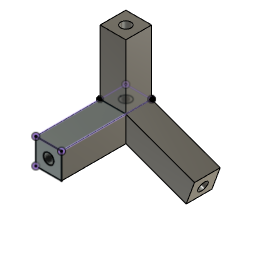
Collin_Corner Connector 2 v1 v1 (Autodesk Fusion 360 design; units mm, degrees)
Autodesk Fusion 360 part; units mm, degrees
sketch "Sketch1" plane through (0, 0, 0) normal (0, 1, 0) x (1, 0, 0)
  line L0 (0, 0) -> (4, 0)
  line L1 (4, 0) -> (4, -4)
  line L2 (4, -4) -> (0, -4)
  line L3 (0, -4) -> (0, 0)
  circle A0 centre (2, -2) radius 0.8
  dimension "d1" = 4
  dimension "d2" = 4
  dimension "d3" = 1.6
  dimension "d4" = 2
  dimension "d5" = 2
  constraint horizontal L0
  constraint vertical L1
  constraint horizontal L2
  constraint vertical L3
  constraint coincident L0.start L3.end
  measures "d1" distance of L1.end L2.end
  measures "d2" distance of L0.end L1.end
  measures "d3" diameter of A0
  measures "d4" distance of L2 A0.centre
  measures "d5" distance of L1 A0.centre
extrude "Extrude1" add sketch "Sketch1" along normal blind 14 makes body 1
sketch "Sketch2" plane through (0, 0, 4) normal (0, 0, 1) x (-1, 0, 0)
  line L0 (0, 0) -> (-4, 0)
  line L1 (-4, 0) -> (-4, -14)
  line L2 (-4, -14) -> (0, -14)
  line L3 (0, -14) -> (0, 0)
  line L4 (-4, -14) -> (0, -14)
  line L5 (0, -14) -> (0, -10)
  line L6 (0, -10) -> (-4, -10)
  line L7 (-4, -10) -> (-4, -14)
  circle A0 centre (-2, -12) radius 0.8
  dimension "d8" = 4
  dimension "d9" = 1.6
  dimension "d10" = 2
  dimension "d11" = 2
  constraint horizontal L4
  constraint vertical L5
  constraint horizontal L6
  constraint vertical L7
  constraint coincident L3 L5.end
  constraint coincident L1.end L2.start
  measures "d8" distance of L4 L6
  measures "d9" diameter of A0
  measures "d10" distance of L5 A0.centre
  measures "d11" distance of L4 A0.centre
extrude "Extrude2" add sketch "Sketch2" along normal blind 10 contours L1 L2 L3 L4 L5 L6 L7 bodies 1
ref_plane "WorkPlane1" through (4, 7, 0) normal (0.939693, 0, -0.34202) x (0, 1, 0)
sketch "Sketch3" plane through (4, 7, 0) normal (0.939693, 0, -0.34202) x (0, 1, 0)
  line L0 (-7, 3.7588) -> (-7, 0)
  line L1 (-7, 0) -> (7, 0)
  line L2 (7, 0) -> (7, 13.1557)
  line L3 (7, 13.1557) -> (3, 13.1557)
  line L4 (3, 13.1557) -> (3, 3.7588)
  line L5 (3, 3.7588) -> (-7, 3.7588)
  line L6 (7, 0) -> (3, 0)
  line L7 (3, 0) -> (3, 3.7588)
  line L8 (3, 3.7588) -> (7, 3.7588)
  line L9 (7, 3.7588) -> (7, 0)
  circle A0 centre (5, 1.7588) radius 0.8
  dimension "d15" = 1.6
  dimension "d16" = 2
  dimension "d17" = 2
  constraint horizontal L6
  constraint vertical L7
  constraint horizontal L8
  constraint vertical L9
  constraint coincident L4.end L5.start
  constraint coincident L1.end L2.start
  measures "d15" diameter of A0
  measures "d16" distance of L8 A0.centre
  measures "d17" distance of L7 A0.centre
extrude "Extrude3" add sketch "Sketch3" along normal blind 10 separate body contours L1 L2 L6 L7 L8 L9 makes body 2
extrude "Extrude4" add 1 faces at (5.1485, 12.0199, 3.1555) along direction (-0.939693, 0, 0.34202) up to surface end surface through (4, 0, 0) normal (1, 0, 0) offset 0 on bodies 2 bodies 2 1
extrude "Extrude5" add sketch "Sketch1" along normal blind 4 from surface at 10 contours A0 bodies 2
